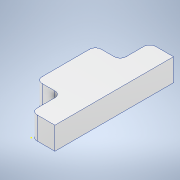
# Autodesk Inventor part: Soporte Riel
Saved by Autodesk Inventor 2020.3 (Build 243373000, 373)
## iProperties
Created: 2020-07-21
Part Number: Soporte Riel
Material: Aluminum 6061
Document SubType Name: Modeling
Designer: juanp
Density: 2.7 g/cm^3
Appearance: Aluminum - Flat
Author: juanp
Autodesk Inventor part; units mm, degrees
ref_plane "YZ Plane" through (0, 0, 0) normal (1, 0, 0) x (0, 1, 0)
ref_plane "XZ Plane" through (0, 0, 0) normal (0, 1, 0) x (-1, 0, 0)
ref_plane "XY Plane" through (0, 0, 0) normal (0, 0, 1) x (1, 0, 0)
sketch "Sketch1" plane through (0, 0, 0) normal (0, 1, 0) x (-1, 0, 0)
  line L0 (0, 0) -> (15, 0) construction
  line L1 (0, 0) -> (20, 0)
  line L2 (20, -5) -> (20, -20)
  line L3 (15, -100) -> (0, -100)
  line L4 (0, -100) -> (0, 0)
  line L5 (20, -50) -> (40.825, -50) construction
  line L6 (35.825, -25) -> (25, -25)
  line L7 (20, -25) -> (20, -75) construction
  line L8 (25, -75) -> (35.825, -75)
  line L9 (40.825, -70) -> (40.825, -30)
  line L10 (40.825, -25) -> (20, -75) construction
  line L11 (20, -25) -> (40.825, -75) construction
  line L12 (40.825, 0) -> (40.825, -9.0602) construction
  line L13 (20, -25) -> (20, -75) construction
  line L14 (20, -80) -> (20, -95)
  arc A0 (20, -5) -> (15, 0) centre (15, -5) ccw
  arc A1 (20, -20) -> (25, -25) centre (25, -20) ccw
  arc A2 (40.825, -30) -> (35.825, -25) centre (35.825, -30) ccw
  arc A3 (35.825, -75) -> (40.825, -70) centre (35.825, -70) ccw
  arc A4 (25, -75) -> (20, -80) centre (25, -80) ccw
  arc A5 (15, -100) -> (20, -95) centre (15, -95) ccw
  point P0 (20, -100)
  point P1 (30.4125, -50)
  dimension "d10" = 40.825
  dimension "d11" = 20
  dimension "d12" = 100
  dimension "d13" = 50
  dimension "d14" = 5
  constraints: 30 end point, 13 point on line, 12 point on circle, 12 tangent, 6 centre point, 6 parallel, 5 equal radius, 4 horizontal, 4 perpendicular, 3 midpoint, 1 collinear, 1 vertical
  measures "d10" distance of L0.start L12.start
  measures "d11" distance of point (20, -100) L3.end
  measures "d12" distance of L1.end point (20, -100)
  measures "d13" distance of L7.end L7.start
  measures "d14" radius of A0
extrude "Extrusion1" add sketch "Sketch1" along normal blind 19.05
sketch "Sketch2" plane through (-20, 0, -20) normal (-1, 0, 0) x (0, 0, 1)
  point P0 (20, 0)
body "Solid1"
